Autodesk Fusion 360 part; units mm, degrees
(part 4 of 6)
extrude "Extrude2" cut sketch "Sketch2" against normal blind 2 contours L4 L5 L6 L7 A0 A1 A2 A3 | A4 L10 L11 A5 A6 L13 L14 A7 | A8 L16 L17 A9 A10 L19 L20 A11 | A12 L22 L23 A13 A14 L25 L26 A15 | A16 L28 L29 A17 A18 L31 L32 A19 | A20 L34 L35 A21 A22 L37 L38 A23 | A24 L40 L41 A25 A26 L43 L44 A27 | A28 L46 L47 A29 A30 L49 L50 A31 | A32 L52 L53 A33 A34 L55 L56 A35 | A36 L58 L59 A37 A38 L61 L62 A39 | A40 L64 L65 A41 A42 L67 L68 A43 | A44 L70 L71 A45 A46 L73 L74 A47 | A48 L76 L77 A49 A50 L79 L80 A51 | A52 L82 L83 A53 A54 L85 L86 A55 | A56 L88 L89 A57 A58 L91 L92 A59 | A60 L94 L95 A61 A62 L97 L98 A63 | A64 L100 L101 A65 A66 L103 L104 A67 | A68 L106 L107 A69 A70 L109 L110 A71 | A72 L112 L113 A73 A74 L115 L116 A75 | A76 L118 L119 A77 A78 L121 L122 A79 | A80 L124 L125 A81 A82 L127 L128 A83 | A84 L130 L131 A85 A86 L133 L134 A87 | A88 L136 L137 A89 A90 L139 L140 A91 | A92 L142 L143 A93 A94 L145 L146 A95 | A96 L148 L149 A97 A98 L151 L152 A99 | A100 L154 L155 A101 A102 L157 L158 A103 | A104 L160 L161 A105 A106 L163 L164 A107 | A108 L166 L167 A109 A110 L169 L170 A111 | A112 L172 L173 A113 A114 L175 L176 A115 | A116 L178 L179 A117 A118 L181 L182 A119 | A120 L184 L185 A121 A122 L187 L188 A123 | A124 L190 L191 A125 A126 L193 L194 A127 | A128 L196 L197 A129 A130 L199 L200 A131 | A132 L202 L203 A133 A134 L205 L206 A135 | A136 L208 L209 A137 A138 L211 L212 A139 | A140 L214 L215 A141 A142 L217 L218 A143 | A144 L220 L221 A145 A146 L223 L224 A147 | A148 L226 L227 A149 A150 L229 L230 A151 | A152 L232 L233 A153 A154 L235 L236 A155 | A156 L238 L239 A157 A158 L241 L242 A159 | A160 L244 L245 A161 A162 L247 L248 A163 | A164 L250 L251 A165 A166 L253 L254 A167 | A168 L256 L257 A169 A170 L259 L260 A171 | A172 L262 L263 A173 A174 L265 L266 A175 | A176 L268 L269 A177 A178 L271 L272 A179 | A180 L274 L275 A181 A182 L277 L278 A183 | A184 L280 L281 A185 A186 L283 L284 A187 | A188 L286 L287 A189 A190 L289 L290 A191 | A192 L292 L293 A193 A194 L295 L296 A195 | A196 L298 L299 A197 A198 L301 L302 A199 | A200 L304 L305 A201 A202 L307 L308 A203 | A204 L310 L311 A205 A206 L313 L314 A207 | A208 L316 L317 A209 A210 L319 L320 A211 | A212 L322 L323 A213 A214 L325 L326 A215 | A216 L328 L329 A217 A218 L331 L332 A219 | A220 L334 L335 A221 A222 L337 L338 A223 | A224 L340 L341 A225 A226 L343 L344 A227 | A228 L346 L347 A229 A230 L349 L350 A231 | A232 L352 L353 A233 A234 L355 L356 A235 | A236 L358 L359 A237 A238 L361 L362 A239 | A240 L364 L365 A241 A242 L367 L368 A243 | A244 L370 L371 A245 A246 L373 L374 A247 | A248 L376 L377 A249 A250 L379 L380 A251 | A252 L382 L383 A253 A254 L385 L386 A255 | A256 L388 L389 A257 A258 L391 L392 A259 | A260 L394 L395 A261 A262 L397 L398 A263 | A264 L400 L401 A265 A266 L403 L404 A267 | A268 L406 L407 A269 A270 L409 L410 A271 | A272 L412 L413 A273 A274 L415 L416 A275 | A276 L418 L419 A277 A278 L421 L422 A279 | A280 L424 L425 A281 A282 L427 L428 A283 | A284 L430 L431 A285 A286 L433 L434 A287 | A288 L436 L437 A289 A290 L439 L440 A291 | A292 L442 L443 A293 A294 L445 L446 A295 | A296 L448 L449 A297 A298 L451 L452 A299 | A300 L454 L455 A301 A302 L457 L458 A303 | A304 L460 L461 A305 A306 L463 L464 A307 | A308 L466 L467 A309 A310 L469 L470 A311 | A312 L472 L473 A313 A314 L475 L476 A315 | A316 L478 L479 A317 A318 L481 L482 A319 | A320 L484 L485 A321 A322 L487 L488 A323 | A324 L490 L491 A325 A326 L493 L494 A327 | A328 L496 L497 A329 A330 L499 L500 A331 | A332 L502 L503 A333 A334 L505 L506 A335 | A336 L508 L509 A337 A338 L511 L512 A339 | A340 L514 L515 A341 A342 L517 L518 A343 | A344 L520 L521 A345 A346 L523 L524 A347 | A348 L526 L527 A349 A350 L529 L530 A351 | A352 L532 L533 A353 A354 L535 L536 A355 | A356 L538 L539 A357 A358 L541 L542 A359 | A360 L544 L545 A361 A362 L547 L548 A363 | A364 L550 L551 A365 A366 L553 L554 A367 | A368 L556 L557 A369 A370 L559 L560 A371 | A372 L562 L563 A373 A374 L565 L566 A375 | A376 L568 L569 A377 A378 L571 L572 A379 | A380 L574 L575 A381 A382 L577 L578 A383 | A384 L580 L581 A385 A386 L583 L584 A387 | A388 L586 L587 A389 A390 L589 L590 A391 | A392 L592 L593 A393 A394 L595 L596 A395 | A396 L598 L599 A397 A398 L601 L602 A399 | A400 L604 L605 A401 A402 L607 L608 A403 | A404 L610 L611 A405 A406 L613 L614 A407 | A408 L616 L617 A409 A410 L619 L620 A411 | A412 L622 L623 A413 A414 L625 L626 A415 | A416 L628 L629 A417 A418 L631 L632 A419 | A420 L634 L635 A421 A422 L637 L638 A423 | A424 L640 L641 A425 A426 L643 L644 A427 | A428 L646 L647 A429 A430 L649 L650 A431 | A432 L652 L653 A433 A434 L655 L656 A435 | A436 L658 L659 A437 A438 L661 L662 A439 | A440 L664 L665 A441 A442 L667 L668 A443 | A444 L670 L671 A445 A446 L673 L674 A447 | A448 L676 L677 A449 A450 L679 L680 A451 | A452 L682 L683 A453 A454 L685 L686 A455 | A456 L688 L689 A457 A458 L691 L692 A459 | A460 L694 L695 A461 A462 L697 L698 A463 | A464 L700 L701 A465 A466 L703 L704 A467 | A468 L706 L707 A469 A470 L709 L710 A471 | A472 L712 L713 A473 A474 L715 L716 A475 | A476 L718 L719 A477 A478 L721 L722 A479 | A480 L724 L725 A481 A482 L727 L728 A483 | A484 L730 L731 A485 A486 L733 L734 A487 | A488 L736 L737 A489 A490 L739 L740 A491 | A492 L742 L743 A493 A494 L745 L746 A495 | A496 L748 L749 A497 A498 L751 L752 A499 | A500 L754 L755 A501 A502 L757 L758 A503 | A504 L760 L761 A505 A506 L763 L764 A507 | A508 L766 L767 A509 A510 L769 L770 A511 | A512 L772 L773 A513 A514 L775 L776 A515 | A516 L778 L779 A517 A518 L781 L782 A519 | A520 L784 L785 A521 A522 L787 L788 A523 | A524 L790 L791 A525 A526 L793 L794 A527 | A528 L796 L797 A529 A530 L799 L800 A531 | A532 L802 L803 A533 A534 L805 L806 A535 | A536 L808 L809 A537 A538 L811 L812 A539 | A540 L814 L815 A541 A542 L817 L818 A543 | A544 L820 L821 A545 A546 L823 L824 A547 | A548 L826 L827 A549 A550 L829 L830 A551 | A552 L832 L833 A553 A554 L835 L836 A555 | A556 L838 L839 A557 A558 L841 L842 A559 | A560 L844 L845 A561 A562 L847 L848 A563 | A564 L850 L851 A565 A566 L853 L854 A567 | A568 L856 L857 A569 A570 L859 L860 A571 | A572 L862 L863 A573 A574 L865 L866 A575 | A576 L868 L869 A577 A578 L871 L872 A579 | A580 L874 L875 A581 A582 L877 L878 A583 | A584 L880 L881 A585 A586 L883 L884 A587 | A588 L886 L887 A589 A590 L889 L890 A591 | A592 L892 L893 A593 A594 L895 L896 A595 | A596 L898 L899 A597 A598 L901 L902 A599 | A600 L904 L905 A601 A602 L907 L908 A603 | A604 L910 L911 A605 A606 L913 L914 A607 | A608 L916 L917 A609 A610 L919 L920 A611 | A612 L922 L923 A613 A614 L925 L926 A615 | A616 L928 L929 A617 A618 L931 L932 A619 | A620 L934 L935 A621 A622 L937 L938 A623 | A624 L940 L941 A625 A626 L943 L944 A627 | A628 L946 L947 A629 A630 L949 L950 A631 | A632 L952 L953 A633 A634 L955 L956 A635 | A636 L958 L959 A637 A638 L961 L962 A639 | A640 L964 L965 A641 A642 L967 L968 A643 | A644 L970 L971 A645 A646 L973 L974 A647 | A648 L976 L977 A649 A650 L979 L980 A651 | A652 L982 L983 A653 A654 L985 L986 A655 | A656 L988 L989 A657 A658 L991 L992 A659 | A660 L994 L995 A661 A662 L997 L998 A663 | A664 L1000 L1001 A665 A666 L1003 L1004 A667 | A668 L1006 L1007 A669 A670 L1009 L1010 A671 | A672 L1012 L1013 A673 A674 L1015 L1016 A675 | A676 L1018 L1019 A677 A678 L1021 L1022 A679 | A680 L1024 L1025 A681 A682 L1027 L1028 A683 | A684 L1030 L1031 A685 A686 L1033 L1034 A687 | A688 L1036 L1037 A689 A690 L1039 L1040 A691 | A692 L1042 L1043 A693 A694 L1045 L1046 A695 | A696 L1048 L1049 A697 A698 L1051 L1052 A699 | A700 L1054 L1055 A701 A702 L1057 L1058 A703 | A704 L1060 L1061 A705 A706 L1063 L1064 A707 | A708 L1066 L1067 A709 A710 L1069 L1070 A711 | A712 L1072 L1073 A713 A714 L1075 L1076 A715 | A716 L1078 L1079 A717 A718 L1081 L1082 A719 | A720 L1084 L1085 A721 A722 L1087 L1088 A723 | A724 L1090 L1091 A725 A726 L1093 L1094 A727 | A728 L1096 L1097 A729 A730 L1099 L1100 A731 | A732 L1102 L1103 A733 A734 L1105 L1106 A735 | A736 L1108 L1109 A737 A738 L1111 L1112 A739 | A740 L1114 L1115 A741 A742 L1117 L1118 A743 | A744 L1120 L1121 A745 A746 L1123 L1124 A747 | A748 L1126 L1127 A749 A750 L1129 L1130 A751 | A752 L1132 L1133 A753 A754 L1135 L1136 A755 | A756 L1138 L1139 A757 A758 L1141 L1142 A759 | A760 L1144 L1145 A761 A762 L1147 L1148 A763 | A764 L1150 L1151 A765 A766 L1153 L1154 A767 | A768 L1156 L1157 A769 A770 L1159 L1160 A771 | A772 L1162 L1163 A773 A774 L1165 L1166 A775 | A776 L1168 L1169 A777 A778 L1171 L1172 A779 | A780 L1174 L1175 A781 A782 L1177 L1178 A783 | A784 L1180 L1181 A785 A786 L1183 L1184 A787 | A788 L1186 L1187 A789 A790 L1189 L1190 A791 | A792 L1192 L1193 A793 A794 L1195 L1196 A795 | A796 L1198 L1199 A797 A798 L1201 L1202 A799 | A800 L1204 L1205 A801 A802 L1207 L1208 A803 | A804 L1210 L1211 A805 A806 L1213 L1214 A807 | A808 L1216 L1217 A809 A810 L1219 L1220 A811 | A812 L1222 L1223 A813 A814 L1225 L1226 A815 | A816 L1228 L1229 A817 A818 L1231 L1232 A819 | A820 L1234 L1235 A821 A822 L1237 L1238 A823 | A824 L1240 L1241 A825 A826 L1243 L1244 A827 | A828 L1246 L1247 A829 A830 L1249 L1250 A831 | A832 L1252 L1253 A833 A834 L1255 L1256 A835 | A836 L1258 L1259 A837 A838 L1261 L1262 A839 | A840 L1264 L1265 A841 A842 L1267 L1268 A843 | A844 L1270 L1271 A845 A846 L1273 L1274 A847 | A848 L1276 L1277 A849 A850 L1279 L1280 A851 | A852 L1282 L1283 A853 A854 L1285 L1286 A855 | A856 L1288 L1289 A857 A858 L1291 L1292 A859 | A860 L1294 L1295 A861 A862 L1297 L1298 A863 | A864 L1300 L1301 A865 A866 L1303 L1304 A867 | A868 L1306 L1307 A869 A870 L1309 L1310 A871 | A872 L1312 L1313 A873 A874 L1315 L1316 A875 | A876 L1318 L1319 A877 A878 L1321 L1322 A879 | A880 L1324 L1325 A881 A882 L1327 L1328 A883 | A884 L1330 L1331 A885 A886 L1333 L1334 A887 | A888 L1336 L1337 A889 A890 L1339 L1340 A891 | A892 L1342 L1343 A893 A894 L1345 L1346 A895 | A896 L1348 L1349 A897 A898 L1351 L1352 A899
fillet "Fillet1" radius 20 4 edges at (-254, 20.5994, 0) (0, 20.5994, -254) (254, 20.5994, 0) (0, 20.5994, 254)
extrude "Extrude3" cut 4 faces at (-165.8917, 18.5994, 164.8333) (-165.8917, 18.5994, -166.95) (165.8917, 18.5994, -164.8333) (164.8333, 18.5994, 165.8917) along direction (0, -1, 0) blind 3
extrude "Extrude4" cut 13 faces at (-98.1083, 18.5994, 164.8333) (2.1083, 18.5994, 164.8333) (93.8917, 18.5994, 164.8333) (164.8333, 18.5994, 93.8917) (164.8333, 18.5994, -2.1083) (164.8333, 18.5994, -98.1083) (93.8917, 18.5994, -171.1667) (-2.1083, 18.5994, -171.1667) (-98.1083, 18.5994, -171.1667) (-164.8333, 18.5994, -98.1083) (-164.8333, 18.5994, -2.1083) (-164.8333, 18.5994, 93.8917) (2.1083, 18.5994, -3.1667) along direction (0, -1, 0) blind 3
extrude "Extrude5" cut 12 faces at (-146.1083, 18.5994, -140.8333) (-118.95, 18.5994, -122.1083) (-97.05, 18.5994, -93.8917) (-69.8917, 18.5994, -75.1667) (-44.8333, 18.5994, -50.1083) (-25.05, 18.5994, -26.1083) (27.1667, 18.5994, 21.8917) (45.8917, 18.5994, 49.05) (73.05, 18.5994, 74.1083) (98.1083, 18.5994, 97.05) (122.1083, 18.5994, 116.8333) (141.8917, 18.5994, 147.1667) along direction (0, -1, 0) blind 3
extrude "Extrude6" cut 12 faces at (141.8917, 18.5994, -140.8333) (123.1667, 18.5994, -117.8917) (93.8917, 18.5994, -94.95) (73.05, 18.5994, -74.1083) (52.225, 18.5994, -51.1667) (27.1667, 18.5994, -26.1083) (-26.1083, 18.5994, 22.95) (-45.8917, 18.5994, 44.8333) (-75.1667, 18.5994, 74.1083) (-98.1083, 18.5994, 97.05) (-118.95, 18.5994, 117.8917) (-146.1083, 18.5994, 147.1667) along direction (0, -1, 0) blind 3
extrude "Extrude7" cut 20 faces at (147.1667, 18.5994, 45.8917) (123.1667, 18.5994, 26.1083) (98.1083, 18.5994, 3.1667) (123.1667, 18.5994, -21.8917) (147.1667, 18.5994, -50.1083) (3.1667, 18.5994, 93.8917) (-20.8333, 18.5994, 117.8917) (-45.8917, 18.5994, 140.8333) (20.8333, 18.5994, 122.1083) (50.1083, 18.5994, 140.8333) (-98.1083, 18.5994, 3.1667) (-117.8917, 18.5994, 27.1667) (-140.8333, 18.5994, 45.8917) (-118.95, 18.5994, -21.8917) (-140.8333, 18.5994, -50.1083) (3.1667, 18.5994, -98.1083) (20.8333, 18.5994, -117.8917) (50.1083, 18.5994, -147.1667) (-20.8333, 18.5994, -122.1083) (-45.8917, 18.5994, -147.1667) along direction (0, -1, 0) blind 3
sketch "Sketch5" plane through (0, 20.5994, 0) normal (0, 1, 0) x (-1, 0, 0)
  line L0 (110.5, -150.325) -> (110.5, -137.675)
  arc A0 (113.675, -134.5) -> (110.5, -137.675) centre (113.675, -137.675) ccw
  line L1 (113.675, -134.5) -> (126.325, -134.5)
  arc A1 (129.5, -137.675) -> (126.325, -134.5) centre (126.325, -137.675) ccw
  line L2 (129.5, -137.675) -> (129.5, -150.325)
  arc A2 (126.325, -153.5) -> (129.5, -150.325) centre (126.325, -150.325) ccw
  line L3 (126.325, -153.5) -> (113.675, -153.5)
  arc A3 (110.5, -150.325) -> (113.675, -153.5) centre (113.675, -150.325) ccw
  line L4 (-9.5, -78.325) -> (-9.5, -65.675)
  arc A4 (-6.325, -62.5) -> (-9.5, -65.675) centre (-6.325, -65.675) ccw
  line L5 (-6.325, -62.5) -> (6.325, -62.5)
  arc A5 (9.5, -65.675) -> (6.325, -62.5) centre (6.325, -65.675) ccw
  line L6 (9.5, -65.675) -> (9.5, -78.325)
  arc A6 (6.325, -81.5) -> (9.5, -78.325) centre (6.325, -78.325) ccw
  line L7 (6.325, -81.5) -> (-6.325, -81.5)
  arc A7 (-9.5, -78.325) -> (-6.325, -81.5) centre (-6.325, -78.325) ccw
  line L8 (-153.5, 41.675) -> (-153.5, 54.325)
  arc A8 (-150.325, 57.5) -> (-153.5, 54.325) centre (-150.325, 54.325) ccw
  line L9 (-150.325, 57.5) -> (-137.675, 57.5)
  arc A9 (-134.5, 54.325) -> (-137.675, 57.5) centre (-137.675, 54.325) ccw
  line L10 (-134.5, 54.325) -> (-134.5, 41.675)
  arc A10 (-137.675, 38.5) -> (-134.5, 41.675) centre (-137.675, 41.675) ccw
  line L11 (-137.675, 38.5) -> (-150.325, 38.5)
  arc A11 (-153.5, 41.675) -> (-150.325, 38.5) centre (-150.325, 41.675) ccw
  line L12 (-81.5, -150.325) -> (-81.5, -137.675)
  arc A12 (-78.325, -134.5) -> (-81.5, -137.675) centre (-78.325, -137.675) ccw
  line L13 (-78.325, -134.5) -> (-65.675, -134.5)
  arc A13 (-62.5, -137.675) -> (-65.675, -134.5) centre (-65.675, -137.675) ccw
  line L14 (-62.5, -137.675) -> (-62.5, -150.325)
  arc A14 (-65.675, -153.5) -> (-62.5, -150.325) centre (-65.675, -150.325) ccw
  line L15 (-65.675, -153.5) -> (-78.325, -153.5)
  arc A15 (-81.5, -150.325) -> (-78.325, -153.5) centre (-78.325, -150.325) ccw
  line L16 (-33.5, -174.325) -> (-33.5, -161.675)
  arc A16 (-30.325, -158.5) -> (-33.5, -161.675) centre (-30.325, -161.675) ccw
  line L17 (-30.325, -158.5) -> (-17.675, -158.5)
  arc A17 (-14.5, -161.675) -> (-17.675, -158.5) centre (-17.675, -161.675) ccw
  line L18 (-14.5, -161.675) -> (-14.5, -174.325)
  arc A18 (-17.675, -177.5) -> (-14.5, -174.325) centre (-17.675, -174.325) ccw
  line L19 (-17.675, -177.5) -> (-30.325, -177.5)
  arc A19 (-33.5, -174.325) -> (-30.325, -177.5) centre (-30.325, -174.325) ccw
  line L20 (38.5, -126.325) -> (38.5, -113.675)
  arc A20 (41.675, -110.5) -> (38.5, -113.675) centre (41.675, -113.675) ccw
  line L21 (41.675, -110.5) -> (54.325, -110.5)
  arc A21 (57.5, -113.675) -> (54.325, -110.5) centre (54.325, -113.675) ccw
  line L22 (57.5, -113.675) -> (57.5, -126.325)
  arc A22 (54.325, -129.5) -> (57.5, -126.325) centre (54.325, -126.325) ccw
  line L23 (54.325, -129.5) -> (41.675, -129.5)
  arc A23 (38.5, -126.325) -> (41.675, -129.5) centre (41.675, -126.325) ccw
  line L24 (62.5, -150.325) -> (62.5, -137.675)
  arc A24 (65.675, -134.5) -> (62.5, -137.675) centre (65.675, -137.675) ccw
  line L25 (65.675, -134.5) -> (78.325, -134.5)
  arc A25 (81.5, -137.675) -> (78.325, -134.5) centre (78.325, -137.675) ccw
  line L26 (81.5, -137.675) -> (81.5, -150.325)
  arc A26 (78.325, -153.5) -> (81.5, -150.325) centre (78.325, -150.325) ccw
  line L27 (78.325, -153.5) -> (65.675, -153.5)
  arc A27 (62.5, -150.325) -> (65.675, -153.5) centre (65.675, -150.325) ccw
  line L28 (134.5, -102.325) -> (134.5, -89.675)
  arc A28 (137.675, -86.5) -> (134.5, -89.675) centre (137.675, -89.675) ccw
  line L29 (137.675, -86.5) -> (150.325, -86.5)
  arc A29 (153.5, -89.675) -> (150.325, -86.5) centre (150.325, -89.675) ccw
  line L30 (153.5, -89.675) -> (153.5, -102.325)
  arc A30 (150.325, -105.5) -> (153.5, -102.325) centre (150.325, -102.325) ccw
  line L31 (150.325, -105.5) -> (137.675, -105.5)
  arc A31 (134.5, -102.325) -> (137.675, -105.5) centre (137.675, -102.325) ccw
  line L32 (-33.5, -6.325) -> (-33.5, 6.325)
  arc A32 (-30.325, 9.5) -> (-33.5, 6.325) centre (-30.325, 6.325) ccw
  line L33 (-30.325, 9.5) -> (-17.675, 9.5)
  arc A33 (-14.5, 6.325) -> (-17.675, 9.5) centre (-17.675, 6.325) ccw
  line L34 (-14.5, 6.325) -> (-14.5, -6.325)
  arc A34 (-17.675, -9.5) -> (-14.5, -6.325) centre (-17.675, -6.325) ccw
  line L35 (-17.675, -9.5) -> (-30.325, -9.5)
  arc A35 (-33.5, -6.325) -> (-30.325, -9.5) centre (-30.325, -6.325) ccw
  line L36 (-105.5, -174.325) -> (-105.5, -161.675)
  arc A36 (-102.325, -158.5) -> (-105.5, -161.675) centre (-102.325, -161.675) ccw
  line L37 (-102.325, -158.5) -> (-89.675, -158.5)
  arc A37 (-86.5, -161.675) -> (-89.675, -158.5) centre (-89.675, -161.675) ccw
  line L38 (-86.5, -161.675) -> (-86.5, -174.325)
  arc A38 (-89.675, -177.5) -> (-86.5, -174.325) centre (-89.675, -174.325) ccw
  line L39 (-89.675, -177.5) -> (-102.325, -177.5)
  arc A39 (-105.5, -174.325) -> (-102.325, -177.5) centre (-102.325, -174.325) ccw
  line L40 (-81.5, -30.325) -> (-81.5, -17.675)
  arc A40 (-78.325, -14.5) -> (-81.5, -17.675) centre (-78.325, -17.675) ccw
  line L41 (-78.325, -14.5) -> (-65.675, -14.5)
  arc A41 (-62.5, -17.675) -> (-65.675, -14.5) centre (-65.675, -17.675) ccw
  line L42 (-62.5, -17.675) -> (-62.5, -30.325)
  arc A42 (-65.675, -33.5) -> (-62.5, -30.325) centre (-65.675, -30.325) ccw
  line L43 (-65.675, -33.5) -> (-78.325, -33.5)
  arc A43 (-81.5, -30.325) -> (-78.325, -33.5) centre (-78.325, -30.325) ccw
  line L44 (134.5, -174.325) -> (134.5, -161.675)
  arc A44 (137.675, -158.5) -> (134.5, -161.675) centre (137.675, -161.675) ccw
  line L45 (137.675, -158.5) -> (150.325, -158.5)
  arc A45 (153.5, -161.675) -> (150.325, -158.5) centre (150.325, -161.675) ccw
  line L46 (153.5, -161.675) -> (153.5, -174.325)
  arc A46 (150.325, -177.5) -> (153.5, -174.325) centre (150.325, -174.325) ccw
  line L47 (150.325, -177.5) -> (137.675, -177.5)
  arc A47 (134.5, -174.325) -> (137.675, -177.5) centre (137.675, -174.325) ccw
  line L48 (158.5, -150.325) -> (158.5, -137.675)
  arc A48 (161.675, -134.5) -> (158.5, -137.675) centre (161.675, -137.675) ccw
  line L49 (161.675, -134.5) -> (174.325, -134.5)
  arc A49 (177.5, -137.675) -> (174.325, -134.5) centre (174.325, -137.675) ccw
  line L50 (177.5, -137.675) -> (177.5, -150.325)
  arc A50 (174.325, -153.5) -> (177.5, -150.325) centre (174.325, -150.325) ccw
  line L51 (174.325, -153.5) -> (161.675, -153.5)
  arc A51 (158.5, -150.325) -> (161.675, -153.5) centre (161.675, -150.325) ccw
  line L52 (110.5, -78.325) -> (110.5, -65.675)
  arc A52 (113.675, -62.5) -> (110.5, -65.675) centre (113.675, -65.675) ccw
  line L53 (113.675, -62.5) -> (126.325, -62.5)
  arc A53 (129.5, -65.675) -> (126.325, -62.5) centre (126.325, -65.675) ccw
  line L54 (129.5, -65.675) -> (129.5, -78.325)
  arc A54 (126.325, -81.5) -> (129.5, -78.325) centre (126.325, -78.325) ccw
  line L55 (126.325, -81.5) -> (113.675, -81.5)
  arc A55 (110.5, -78.325) -> (113.675, -81.5) centre (113.675, -78.325) ccw
  line L56 (62.5, -126.325) -> (62.5, -113.675)
  arc A56 (65.675, -110.5) -> (62.5, -113.675) centre (65.675, -113.675) ccw
  line L57 (65.675, -110.5) -> (78.325, -110.5)
  arc A57 (81.5, -113.675) -> (78.325, -110.5) centre (78.325, -113.675) ccw
  line L58 (81.5, -113.675) -> (81.5, -126.325)
  arc A58 (78.325, -129.5) -> (81.5, -126.325) centre (78.325, -126.325) ccw
  line L59 (78.325, -129.5) -> (65.675, -129.5)
  arc A59 (62.5, -126.325) -> (65.675, -129.5) centre (65.675, -126.325) ccw
  line L60 (62.5, -102.325) -> (62.5, -89.675)
  arc A60 (65.675, -86.5) -> (62.5, -89.675) centre (65.675, -89.675) ccw
  line L61 (65.675, -86.5) -> (78.325, -86.5)
  arc A61 (81.5, -89.675) -> (78.325, -86.5) centre (78.325, -89.675) ccw
  line L62 (81.5, -89.675) -> (81.5, -102.325)
  arc A62 (78.325, -105.5) -> (81.5, -102.325) centre (78.325, -102.325) ccw
  line L63 (78.325, -105.5) -> (65.675, -105.5)
  arc A63 (62.5, -102.325) -> (65.675, -105.5) centre (65.675, -102.325) ccw
  line L64 (14.5, -30.325) -> (14.5, -17.675)
  arc A64 (17.675, -14.5) -> (14.5, -17.675) centre (17.675, -17.675) ccw
  line L65 (17.675, -14.5) -> (30.325, -14.5)
  arc A65 (33.5, -17.675) -> (30.325, -14.5) centre (30.325, -17.675) ccw
  line L66 (33.5, -17.675) -> (33.5, -30.325)
  arc A66 (30.325, -33.5) -> (33.5, -30.325) centre (30.325, -30.325) ccw
  line L67 (30.325, -33.5) -> (17.675, -33.5)
  arc A67 (14.5, -30.325) -> (17.675, -33.5) centre (17.675, -30.325) ccw
  line L68 (110.5, -6.325) -> (110.5, 6.325)
  arc A68 (113.675, 9.5) -> (110.5, 6.325) centre (113.675, 6.325) ccw
  line L69 (113.675, 9.5) -> (126.325, 9.5)
  arc A69 (129.5, 6.325) -> (126.325, 9.5) centre (126.325, 6.325) ccw
  line L70 (129.5, 6.325) -> (129.5, -6.325)
  arc A70 (126.325, -9.5) -> (129.5, -6.325) centre (126.325, -6.325) ccw
  line L71 (126.325, -9.5) -> (113.675, -9.5)
  arc A71 (110.5, -6.325) -> (113.675, -9.5) centre (113.675, -6.325) ccw
  line L72 (110.5, 17.675) -> (110.5, 30.325)
  arc A72 (113.675, 33.5) -> (110.5, 30.325) centre (113.675, 30.325) ccw
  line L73 (113.675, 33.5) -> (126.325, 33.5)
  arc A73 (129.5, 30.325) -> (126.325, 33.5) centre (126.325, 30.325) ccw
  line L74 (129.5, 30.325) -> (129.5, 17.675)
  arc A74 (126.325, 14.5) -> (129.5, 17.675) centre (126.325, 17.675) ccw
  line L75 (126.325, 14.5) -> (113.675, 14.5)
  arc A75 (110.5, 17.675) -> (113.675, 14.5) centre (113.675, 17.675) ccw
  line L76 (110.5, 41.675) -> (110.5, 54.325)
  arc A76 (113.675, 57.5) -> (110.5, 54.325) centre (113.675, 54.325) ccw
  line L77 (113.675, 57.5) -> (126.325, 57.5)
  arc A77 (129.5, 54.325) -> (126.325, 57.5) centre (126.325, 54.325) ccw
  line L78 (129.5, 54.325) -> (129.5, 41.675)
  arc A78 (126.325, 38.5) -> (129.5, 41.675) centre (126.325, 41.675) ccw
  line L79 (126.325, 38.5) -> (113.675, 38.5)
  arc A79 (110.5, 41.675) -> (113.675, 38.5) centre (113.675, 41.675) ccw
  line L80 (110.5, 65.675) -> (110.5, 78.325)
  arc A80 (113.675, 81.5) -> (110.5, 78.325) centre (113.675, 78.325) ccw
  line L81 (113.675, 81.5) -> (126.325, 81.5)
  arc A81 (129.5, 78.325) -> (126.325, 81.5) centre (126.325, 78.325) ccw
  line L82 (129.5, 78.325) -> (129.5, 65.675)
  arc A82 (126.325, 62.5) -> (129.5, 65.675) centre (126.325, 65.675) ccw
  line L83 (126.325, 62.5) -> (113.675, 62.5)
  arc A83 (110.5, 65.675) -> (113.675, 62.5) centre (113.675, 65.675) ccw
  line L84 (110.5, 89.675) -> (110.5, 102.325)
  arc A84 (113.675, 105.5) -> (110.5, 102.325) centre (113.675, 102.325) ccw
  line L85 (113.675, 105.5) -> (126.325, 105.5)
  arc A85 (129.5, 102.325) -> (126.325, 105.5) centre (126.325, 102.325) ccw
  line L86 (129.5, 102.325) -> (129.5, 89.675)
  arc A86 (126.325, 86.5) -> (129.5, 89.675) centre (126.325, 89.675) ccw
  line L87 (126.325, 86.5) -> (113.675, 86.5)
  arc A87 (110.5, 89.675) -> (113.675, 86.5) centre (113.675, 89.675) ccw
  line L88 (110.5, 113.675) -> (110.5, 126.325)
  arc A88 (113.675, 129.5) -> (110.5, 126.325) centre (113.675, 126.325) ccw
  line L89 (113.675, 129.5) -> (126.325, 129.5)
  arc A89 (129.5, 126.325) -> (126.325, 129.5) centre (126.325, 126.325) ccw
  line L90 (129.5, 126.325) -> (129.5, 113.675)
  arc A90 (126.325, 110.5) -> (129.5, 113.675) centre (126.325, 113.675) ccw
  line L91 (126.325, 110.5) -> (113.675, 110.5)
  arc A91 (110.5, 113.675) -> (113.675, 110.5) centre (113.675, 113.675) ccw
  line L92 (110.5, 137.675) -> (110.5, 150.325)
  arc A92 (113.675, 153.5) -> (110.5, 150.325) centre (113.675, 150.325) ccw
  line L93 (113.675, 153.5) -> (126.325, 153.5)
  arc A93 (129.5, 150.325) -> (126.325, 153.5) centre (126.325, 150.325) ccw
  line L94 (129.5, 150.325) -> (129.5, 137.675)
  arc A94 (126.325, 134.5) -> (129.5, 137.675) centre (126.325, 137.675) ccw
  line L95 (126.325, 134.5) -> (113.675, 134.5)
  arc A95 (110.5, 137.675) -> (113.675, 134.5) centre (113.675, 137.675) ccw
  line L96 (110.5, 161.675) -> (110.5, 174.325)
  arc A96 (113.675, 177.5) -> (110.5, 174.325) centre (113.675, 174.325) ccw
  line L97 (113.675, 177.5) -> (126.325, 177.5)
  arc A97 (129.5, 174.325) -> (126.325, 177.5) centre (126.325, 174.325) ccw
  line L98 (129.5, 174.325) -> (129.5, 161.675)
  arc A98 (126.325, 158.5) -> (129.5, 161.675) centre (126.325, 161.675) ccw
  line L99 (126.325, 158.5) -> (113.675, 158.5)
  arc A99 (110.5, 161.675) -> (113.675, 158.5) centre (113.675, 161.675) ccw
  line L100 (38.5, -6.325) -> (38.5, 6.325)
  arc A100 (41.675, 9.5) -> (38.5, 6.325) centre (41.675, 6.325) ccw
  line L101 (41.675, 9.5) -> (54.325, 9.5)
  arc A101 (57.5, 6.325) -> (54.325, 9.5) centre (54.325, 6.325) ccw
  line L102 (57.5, 6.325) -> (57.5, -6.325)
  arc A102 (54.325, -9.5) -> (57.5, -6.325) centre (54.325, -6.325) ccw
  line L103 (54.325, -9.5) -> (41.675, -9.5)
  arc A103 (38.5, -6.325) -> (41.675, -9.5) centre (41.675, -6.325) ccw
  line L104 (38.5, 17.675) -> (38.5, 30.325)
  arc A104 (41.675, 33.5) -> (38.5, 30.325) centre (41.675, 30.325) ccw
  line L105 (41.675, 33.5) -> (54.325, 33.5)
  arc A105 (57.5, 30.325) -> (54.325, 33.5) centre (54.325, 30.325) ccw
  line L106 (57.5, 30.325) -> (57.5, 17.675)
  arc A106 (54.325, 14.5) -> (57.5, 17.675) centre (54.325, 17.675) ccw
  line L107 (54.325, 14.5) -> (41.675, 14.5)
  arc A107 (38.5, 17.675) -> (41.675, 14.5) centre (41.675, 17.675) ccw
  line L108 (38.5, 41.675) -> (38.5, 54.325)
  arc A108 (41.675, 57.5) -> (38.5, 54.325) centre (41.675, 54.325) ccw
  line L109 (41.675, 57.5) -> (54.325, 57.5)
  arc A109 (57.5, 54.325) -> (54.325, 57.5) centre (54.325, 54.325) ccw
  line L110 (57.5, 54.325) -> (57.5, 41.675)
  arc A110 (54.325, 38.5) -> (57.5, 41.675) centre (54.325, 41.675) ccw
  line L111 (54.325, 38.5) -> (41.675, 38.5)
  arc A111 (38.5, 41.675) -> (41.675, 38.5) centre (41.675, 41.675) ccw
  line L112 (38.5, 65.675) -> (38.5, 78.325)
  arc A112 (41.675, 81.5) -> (38.5, 78.325) centre (41.675, 78.325) ccw
  line L113 (41.675, 81.5) -> (54.325, 81.5)
  arc A113 (57.5, 78.325) -> (54.325, 81.5) centre (54.325, 78.325) ccw
  line L114 (57.5, 78.325) -> (57.5, 65.675)
  arc A114 (54.325, 62.5) -> (57.5, 65.675) centre (54.325, 65.675) ccw
  line L115 (54.325, 62.5) -> (41.675, 62.5)
  arc A115 (38.5, 65.675) -> (41.675, 62.5) centre (41.675, 65.675) ccw
  line L116 (14.5, 89.675) -> (14.5, 102.325)
  arc A116 (17.675, 105.5) -> (14.5, 102.325) centre (17.675, 102.325) ccw
  line L117 (17.675, 105.5) -> (30.325, 105.5)
  arc A117 (33.5, 102.325) -> (30.325, 105.5) centre (30.325, 102.325) ccw
  line L118 (33.5, 102.325) -> (33.5, 89.675)
  arc A118 (30.325, 86.5) -> (33.5, 89.675) centre (30.325, 89.675) ccw
  line L119 (30.325, 86.5) -> (17.675, 86.5)
  arc A119 (14.5, 89.675) -> (17.675, 86.5) centre (17.675, 89.675) ccw
  line L120 (14.5, 113.675) -> (14.5, 126.325)
  arc A120 (17.675, 129.5) -> (14.5, 126.325) centre (17.675, 126.325) ccw
  line L121 (17.675, 129.5) -> (30.325, 129.5)
  arc A121 (33.5, 126.325) -> (30.325, 129.5) centre (30.325, 126.325) ccw
  line L122 (33.5, 126.325) -> (33.5, 113.675)
  arc A122 (30.325, 110.5) -> (33.5, 113.675) centre (30.325, 113.675) ccw
  line L123 (30.325, 110.5) -> (17.675, 110.5)
  arc A123 (14.5, 113.675) -> (17.675, 110.5) centre (17.675, 113.675) ccw
  line L124 (14.5, 137.675) -> (14.5, 150.325)
  arc A124 (17.675, 153.5) -> (14.5, 150.325) centre (17.675, 150.325) ccw
  line L125 (17.675, 153.5) -> (30.325, 153.5)
  arc A125 (33.5, 150.325) -> (30.325, 153.5) centre (30.325, 150.325) ccw
  line L126 (33.5, 150.325) -> (33.5, 137.675)
  arc A126 (30.325, 134.5) -> (33.5, 137.675) centre (30.325, 137.675) ccw
  line L127 (30.325, 134.5) -> (17.675, 134.5)
  arc A127 (14.5, 137.675) -> (17.675, 134.5) centre (17.675, 137.675) ccw
  line L128 (-9.5, 161.675) -> (-9.5, 174.325)
  arc A128 (-6.325, 177.5) -> (-9.5, 174.325) centre (-6.325, 174.325) ccw
  line L129 (-6.325, 177.5) -> (6.325, 177.5)
  arc A129 (9.5, 174.325) -> (6.325, 177.5) centre (6.325, 174.325) ccw
  line L130 (9.5, 174.325) -> (9.5, 161.675)
  arc A130 (6.325, 158.5) -> (9.5, 161.675) centre (6.325, 161.675) ccw
  line L131 (6.325, 158.5) -> (-6.325, 158.5)
  arc A131 (-9.5, 161.675) -> (-6.325, 158.5) centre (-6.325, 161.675) ccw
  line L132 (-105.5, 17.675) -> (-105.5, 30.325)
  arc A132 (-102.325, 33.5) -> (-105.5, 30.325) centre (-102.325, 30.325) ccw
  line L133 (-102.325, 33.5) -> (-89.675, 33.5)
  arc A133 (-86.5, 30.325) -> (-89.675, 33.5) centre (-89.675, 30.325) ccw
  line L134 (-86.5, 30.325) -> (-86.5, 17.675)
  arc A134 (-89.675, 14.5) -> (-86.5, 17.675) centre (-89.675, 17.675) ccw
  line L135 (-89.675, 14.5) -> (-102.325, 14.5)
  arc A135 (-105.5, 17.675) -> (-102.325, 14.5) centre (-102.325, 17.675) ccw
  line L136 (-129.5, 41.675) -> (-129.5, 54.325)
  arc A136 (-126.325, 57.5) -> (-129.5, 54.325) centre (-126.325, 54.325) ccw
  line L137 (-126.325, 57.5) -> (-113.675, 57.5)
  arc A137 (-110.5, 54.325) -> (-113.675, 57.5) centre (-113.675, 54.325) ccw
  line L138 (-110.5, 54.325) -> (-110.5, 41.675)
  arc A138 (-113.675, 38.5) -> (-110.5, 41.675) centre (-113.675, 41.675) ccw
  line L139 (-113.675, 38.5) -> (-126.325, 38.5)
  arc A139 (-129.5, 41.675) -> (-126.325, 38.5) centre (-126.325, 41.675) ccw
  line L140 (-153.5, -30.325) -> (-153.5, -17.675)
  arc A140 (-150.325, -14.5) -> (-153.5, -17.675) centre (-150.325, -17.675) ccw
  line L141 (-150.325, -14.5) -> (-137.675, -14.5)
  arc A141 (-134.5, -17.675) -> (-137.675, -14.5) centre (-137.675, -17.675) ccw
  line L142 (-134.5, -17.675) -> (-134.5, -30.325)
  arc A142 (-137.675, -33.5) -> (-134.5, -30.325) centre (-137.675, -30.325) ccw
  line L143 (-137.675, -33.5) -> (-150.325, -33.5)
  arc A143 (-153.5, -30.325) -> (-150.325, -33.5) centre (-150.325, -30.325) ccw
  line L144 (-177.5, 17.675) -> (-177.5, 30.325)
  arc A144 (-174.325, 33.5) -> (-177.5, 30.325) centre (-174.325, 30.325) ccw
  line L145 (-174.325, 33.5) -> (-161.675, 33.5)
  arc A145 (-158.5, 30.325) -> (-161.675, 33.5) centre (-161.675, 30.325) ccw
  line L146 (-158.5, 30.325) -> (-158.5, 17.675)
  arc A146 (-161.675, 14.5) -> (-158.5, 17.675) centre (-161.675, 17.675) ccw
  line L147 (-161.675, 14.5) -> (-174.325, 14.5)
  arc A147 (-177.5, 17.675) -> (-174.325, 14.5) centre (-174.325, 17.675) ccw
  line L148 (-9.5, -174.325) -> (-9.5, -161.675)
  arc A148 (-6.325, -158.5) -> (-9.5, -161.675) centre (-6.325, -161.675) ccw
  line L149 (-6.325, -158.5) -> (6.325, -158.5)
  arc A149 (9.5, -161.675) -> (6.325, -158.5) centre (6.325, -161.675) ccw
  line L150 (9.5, -161.675) -> (9.5, -174.325)
  arc A150 (6.325, -177.5) -> (9.5, -174.325) centre (6.325, -174.325) ccw
  line L151 (6.325, -177.5) -> (-6.325, -177.5)
  arc A151 (-9.5, -174.325) -> (-6.325, -177.5) centre (-6.325, -174.325) ccw
  line L152 (-33.5, -126.325) -> (-33.5, -113.675)
  arc A152 (-30.325, -110.5) -> (-33.5, -113.675) centre (-30.325, -113.675) ccw
  line L153 (-30.325, -110.5) -> (-17.675, -110.5)
  arc A153 (-14.5, -113.675) -> (-17.675, -110.5) centre (-17.675, -113.675) ccw
  line L154 (-14.5, -113.675) -> (-14.5, -126.325)
  arc A154 (-17.675, -129.5) -> (-14.5, -126.325) centre (-17.675, -126.325) ccw
  line L155 (-17.675, -129.5) -> (-30.325, -129.5)
  arc A155 (-33.5, -126.325) -> (-30.325, -129.5) centre (-30.325, -126.325) ccw
  line L156 (-81.5, -78.325) -> (-81.5, -65.675)
  arc A156 (-78.325, -62.5) -> (-81.5, -65.675) centre (-78.325, -65.675) ccw
  line L157 (-78.325, -62.5) -> (-65.675, -62.5)
  arc A157 (-62.5, -65.675) -> (-65.675, -62.5) centre (-65.675, -65.675) ccw
  line L158 (-62.5, -65.675) -> (-62.5, -78.325)
  arc A158 (-65.675, -81.5) -> (-62.5, -78.325) centre (-65.675, -78.325) ccw
  line L159 (-65.675, -81.5) -> (-78.325, -81.5)
  arc A159 (-81.5, -78.325) -> (-78.325, -81.5) centre (-78.325, -78.325) ccw
  line L160 (-153.5, -174.325) -> (-153.5, -161.675)
  arc A160 (-150.325, -158.5) -> (-153.5, -161.675) centre (-150.325, -161.675) ccw
  line L161 (-150.325, -158.5) -> (-137.675, -158.5)
  arc A161 (-134.5, -161.675) -> (-137.675, -158.5) centre (-137.675, -161.675) ccw
  line L162 (-134.5, -161.675) -> (-134.5, -174.325)
  arc A162 (-137.675, -177.5) -> (-134.5, -174.325) centre (-137.675, -174.325) ccw
  line L163 (-137.675, -177.5) -> (-150.325, -177.5)
  arc A163 (-153.5, -174.325) -> (-150.325, -177.5) centre (-150.325, -174.325) ccw
  line L164 (-129.5, -150.325) -> (-129.5, -137.675)
  arc A164 (-126.325, -134.5) -> (-129.5, -137.675) centre (-126.325, -137.675) ccw
  line L165 (-126.325, -134.5) -> (-113.675, -134.5)
  arc A165 (-110.5, -137.675) -> (-113.675, -134.5) centre (-113.675, -137.675) ccw
  line L166 (-110.5, -137.675) -> (-110.5, -150.325)
  arc A166 (-113.675, -153.5) -> (-110.5, -150.325) centre (-113.675, -150.325) ccw
  line L167 (-113.675, -153.5) -> (-126.325, -153.5)
  arc A167 (-129.5, -150.325) -> (-126.325, -153.5) centre (-126.325, -150.325) ccw
  line L168 (-177.5, -102.325) -> (-177.5, -89.675)
  arc A168 (-174.325, -86.5) -> (-177.5, -89.675) centre (-174.325, -89.675) ccw
  line L169 (-174.325, -86.5) -> (-161.675, -86.5)
  arc A169 (-158.5, -89.675) -> (-161.675, -86.5) centre (-161.675, -89.675) ccw
  line L170 (-158.5, -89.675) -> (-158.5, -102.325)
  arc A170 (-161.675, -105.5) -> (-158.5, -102.325) centre (-161.675, -102.325) ccw
  line L171 (-161.675, -105.5) -> (-174.325, -105.5)
  arc A171 (-177.5, -102.325) -> (-174.325, -105.5) centre (-174.325, -102.325) ccw
  line L172 (-153.5, -78.325) -> (-153.5, -65.675)
  arc A172 (-150.325, -62.5) -> (-153.5, -65.675) centre (-150.325, -65.675) ccw
  line L173 (-150.325, -62.5) -> (-137.675, -62.5)
  arc A173 (-134.5, -65.675) -> (-137.675, -62.5) centre (-137.675, -65.675) ccw
  line L174 (-134.5, -65.675) -> (-134.5, -78.325)
  arc A174 (-137.675, -81.5) -> (-134.5, -78.325) centre (-137.675, -78.325) ccw
  line L175 (-137.675, -81.5) -> (-150.325, -81.5)
  arc A175 (-153.5, -78.325) -> (-150.325, -81.5) centre (-150.325, -78.325) ccw
  line L176 (-33.5, 41.675) -> (-33.5, 54.325)
  arc A176 (-30.325, 57.5) -> (-33.5, 54.325) centre (-30.325, 54.325) ccw
  line L177 (-30.325, 57.5) -> (-17.675, 57.5)
  arc A177 (-14.5, 54.325) -> (-17.675, 57.5) centre (-17.675, 54.325) ccw
  line L178 (-14.5, 54.325) -> (-14.5, 41.675)
  arc A178 (-17.675, 38.5) -> (-14.5, 41.675) centre (-17.675, 41.675) ccw
  line L179 (-17.675, 38.5) -> (-30.325, 38.5)
  arc A179 (-33.5, 41.675) -> (-30.325, 38.5) centre (-30.325, 41.675) ccw
  line L180 (-105.5, 65.675) -> (-105.5, 78.325)
  arc A180 (-102.325, 81.5) -> (-105.5, 78.325) centre (-102.325, 78.325) ccw
  line L181 (-102.325, 81.5) -> (-89.675, 81.5)
  arc A181 (-86.5, 78.325) -> (-89.675, 81.5) centre (-89.675, 78.325) ccw
  line L182 (-86.5, 78.325) -> (-86.5, 65.675)
  arc A182 (-89.675, 62.5) -> (-86.5, 65.675) centre (-89.675, 65.675) ccw
  line L183 (-89.675, 62.5) -> (-102.325, 62.5)
  arc A183 (-105.5, 65.675) -> (-102.325, 62.5) centre (-102.325, 65.675) ccw
  line L184 (-177.5, 89.675) -> (-177.5, 102.325)
  arc A184 (-174.325, 105.5) -> (-177.5, 102.325) centre (-174.325, 102.325) ccw
  line L185 (-174.325, 105.5) -> (-161.675, 105.5)
  arc A185 (-158.5, 102.325) -> (-161.675, 105.5) centre (-161.675, 102.325) ccw
  line L186 (-158.5, 102.325) -> (-158.5, 89.675)
  arc A186 (-161.675, 86.5) -> (-158.5, 89.675) centre (-161.675, 89.675) ccw
  line L187 (-161.675, 86.5) -> (-174.325, 86.5)
  arc A187 (-177.5, 89.675) -> (-174.325, 86.5) centre (-174.325, 89.675) ccw
  line L188 (-81.5, 89.675) -> (-81.5, 102.325)
  arc A188 (-78.325, 105.5) -> (-81.5, 102.325) centre (-78.325, 102.325) ccw
  line L189 (-78.325, 105.5) -> (-65.675, 105.5)
  arc A189 (-62.5, 102.325) -> (-65.675, 105.5) centre (-65.675, 102.325) ccw
  line L190 (-62.5, 102.325) -> (-62.5, 89.675)
  arc A190 (-65.675, 86.5) -> (-62.5, 89.675) centre (-65.675, 89.675) ccw
  line L191 (-65.675, 86.5) -> (-78.325, 86.5)
  arc A191 (-81.5, 89.675) -> (-78.325, 86.5) centre (-78.325, 89.675) ccw
  line L192 (-153.5, 113.675) -> (-153.5, 126.325)
  arc A192 (-150.325, 129.5) -> (-153.5, 126.325) centre (-150.325, 126.325) ccw
  line L193 (-150.325, 129.5) -> (-137.675, 129.5)
  arc A193 (-134.5, 126.325) -> (-137.675, 129.5) centre (-137.675, 126.325) ccw
  line L194 (-134.5, 126.325) -> (-134.5, 113.675)
  arc A194 (-137.675, 110.5) -> (-134.5, 113.675) centre (-137.675, 113.675) ccw
  line L195 (-137.675, 110.5) -> (-150.325, 110.5)
  arc A195 (-153.5, 113.675) -> (-150.325, 110.5) centre (-150.325, 113.675) ccw
  line L196 (-57.5, 113.675) -> (-57.5, 126.325)
  arc A196 (-54.325, 129.5) -> (-57.5, 126.325) centre (-54.325, 126.325) ccw
  line L197 (-54.325, 129.5) -> (-41.675, 129.5)
  arc A197 (-38.5, 126.325) -> (-41.675, 129.5) centre (-41.675, 126.325) ccw
  line L198 (-38.5, 126.325) -> (-38.5, 113.675)
  arc A198 (-41.675, 110.5) -> (-38.5, 113.675) centre (-41.675, 113.675) ccw
  line L199 (-41.675, 110.5) -> (-54.325, 110.5)
  arc A199 (-57.5, 113.675) -> (-54.325, 110.5) centre (-54.325, 113.675) ccw
  line L200 (-129.5, 137.675) -> (-129.5, 150.325)
  arc A200 (-126.325, 153.5) -> (-129.5, 150.325) centre (-126.325, 150.325) ccw
  line L201 (-126.325, 153.5) -> (-113.675, 153.5)
  arc A201 (-110.5, 150.325) -> (-113.675, 153.5) centre (-113.675, 150.325) ccw
  line L202 (-110.5, 150.325) -> (-110.5, 137.675)
  arc A202 (-113.675, 134.5) -> (-110.5, 137.675) centre (-113.675, 137.675) ccw
  line L203 (-113.675, 134.5) -> (-126.325, 134.5)
  arc A203 (-129.5, 137.675) -> (-126.325, 134.5) centre (-126.325, 137.675) ccw
  line L204 (-33.5, 137.675) -> (-33.5, 150.325)
  arc A204 (-30.325, 153.5) -> (-33.5, 150.325) centre (-30.325, 150.325) ccw
  line L205 (-30.325, 153.5) -> (-17.675, 153.5)
  arc A205 (-14.5, 150.325) -> (-17.675, 153.5) centre (-17.675, 150.325) ccw
  line L206 (-14.5, 150.325) -> (-14.5, 137.675)
  arc A206 (-17.675, 134.5) -> (-14.5, 137.675) centre (-17.675, 137.675) ccw
  line L207 (-17.675, 134.5) -> (-30.325, 134.5)
  arc A207 (-33.5, 137.675) -> (-30.325, 134.5) centre (-30.325, 137.675) ccw
  line L208 (-105.5, 161.675) -> (-105.5, 174.325)
  arc A208 (-102.325, 177.5) -> (-105.5, 174.325) centre (-102.325, 174.325) ccw
  line L209 (-102.325, 177.5) -> (-89.675, 177.5)
  arc A209 (-86.5, 174.325) -> (-89.675, 177.5) centre (-89.675, 174.325) ccw
  line L210 (-86.5, 174.325) -> (-86.5, 161.675)
  arc A210 (-89.675, 158.5) -> (-86.5, 161.675) centre (-89.675, 161.675) ccw
  line L211 (-89.675, 158.5) -> (-102.325, 158.5)
  arc A211 (-105.5, 161.675) -> (-102.325, 158.5) centre (-102.325, 161.675) ccw
  line L212 (86.5, -174.325) -> (86.5, -161.675)
  arc A212 (89.675, -158.5) -> (86.5, -161.675) centre (89.675, -161.675) ccw
  line L213 (89.675, -158.5) -> (102.325, -158.5)
  arc A213 (105.5, -161.675) -> (102.325, -158.5) centre (102.325, -161.675) ccw
  line L214 (105.5, -161.675) -> (105.5, -174.325)
  arc A214 (102.325, -177.5) -> (105.5, -174.325) centre (102.325, -174.325) ccw
  line L215 (102.325, -177.5) -> (89.675, -177.5)
  arc A215 (86.5, -174.325) -> (89.675, -177.5) centre (89.675, -174.325) ccw
  line L216 (134.5, -126.325) -> (134.5, -113.675)
  arc A216 (137.675, -110.5) -> (134.5, -113.675) centre (137.675, -113.675) ccw
  line L217 (137.675, -110.5) -> (150.325, -110.5)
  arc A217 (153.5, -113.675) -> (150.325, -110.5) centre (150.325, -113.675) ccw
  line L218 (153.5, -113.675) -> (153.5, -126.325)
  arc A218 (150.325, -129.5) -> (153.5, -126.325) centre (150.325, -126.325) ccw
  line L219 (150.325, -129.5) -> (137.675, -129.5)
  arc A219 (134.5, -126.325) -> (137.675, -129.5) centre (137.675, -126.325) ccw
  line L220 (86.5, -54.325) -> (86.5, -41.675)
  arc A220 (89.675, -38.5) -> (86.5, -41.675) centre (89.675, -41.675) ccw
  line L221 (89.675, -38.5) -> (102.325, -38.5)
  arc A221 (105.5, -41.675) -> (102.325, -38.5) centre (102.325, -41.675) ccw
  line L222 (105.5, -41.675) -> (105.5, -54.325)
  arc A222 (102.325, -57.5) -> (105.5, -54.325) centre (102.325, -54.325) ccw
  line L223 (102.325, -57.5) -> (89.675, -57.5)
  arc A223 (86.5, -54.325) -> (89.675, -57.5) centre (89.675, -54.325) ccw
  line L224 (-177.5, 41.675) -> (-177.5, 54.325)
  arc A224 (-174.325, 57.5) -> (-177.5, 54.325) centre (-174.325, 54.325) ccw
  line L225 (-174.325, 57.5) -> (-161.675, 57.5)
  arc A225 (-158.5, 54.325) -> (-161.675, 57.5) centre (-161.675, 54.325) ccw
  line L226 (-158.5, 54.325) -> (-158.5, 41.675)
  arc A226 (-161.675, 38.5) -> (-158.5, 41.675) centre (-161.675, 41.675) ccw
  line L227 (-161.675, 38.5) -> (-174.325, 38.5)
  arc A227 (-177.5, 41.675) -> (-174.325, 38.5) centre (-174.325, 41.675) ccw
  line L228 (110.5, -54.325) -> (110.5, -41.675)
  arc A228 (113.675, -38.5) -> (110.5, -41.675) centre (113.675, -41.675) ccw
  line L229 (113.675, -38.5) -> (126.325, -38.5)
  arc A229 (129.5, -41.675) -> (126.325, -38.5) centre (126.325, -41.675) ccw
  line L230 (129.5, -41.675) -> (129.5, -54.325)
  arc A230 (126.325, -57.5) -> (129.5, -54.325) centre (126.325, -54.325) ccw
  line L231 (126.325, -57.5) -> (113.675, -57.5)
  arc A231 (110.5, -54.325) -> (113.675, -57.5) centre (113.675, -54.325) ccw
  line L232 (158.5, -126.325) -> (158.5, -113.675)
  arc A232 (161.675, -110.5) -> (158.5, -113.675) centre (161.675, -113.675) ccw
  line L233 (161.675, -110.5) -> (174.325, -110.5)
  arc A233 (177.5, -113.675) -> (174.325, -110.5) centre (174.325, -113.675) ccw
  line L234 (177.5, -113.675) -> (177.5, -126.325)
  arc A234 (174.325, -129.5) -> (177.5, -126.325) centre (174.325, -126.325) ccw
  line L235 (174.325, -129.5) -> (161.675, -129.5)
  arc A235 (158.5, -126.325) -> (161.675, -129.5) centre (161.675, -126.325) ccw
  line L236 (110.5, -174.325) -> (110.5, -161.675)
  arc A236 (113.675, -158.5) -> (110.5, -161.675) centre (113.675, -161.675) ccw
  line L237 (113.675, -158.5) -> (126.325, -158.5)
  arc A237 (129.5, -161.675) -> (126.325, -158.5) centre (126.325, -161.675) ccw
  line L238 (129.5, -161.675) -> (129.5, -174.325)
  arc A238 (126.325, -177.5) -> (129.5, -174.325) centre (126.325, -174.325) ccw
  line L239 (126.325, -177.5) -> (113.675, -177.5)
  arc A239 (110.5, -174.325) -> (113.675, -177.5) centre (113.675, -174.325) ccw
  line L240 (-81.5, 161.675) -> (-81.5, 174.325)
  arc A240 (-78.325, 177.5) -> (-81.5, 174.325) centre (-78.325, 174.325) ccw
  line L241 (-78.325, 177.5) -> (-65.675, 177.5)
  arc A241 (-62.5, 174.325) -> (-65.675, 177.5) centre (-65.675, 174.325) ccw
  line L242 (-62.5, 174.325) -> (-62.5, 161.675)
  arc A242 (-65.675, 158.5) -> (-62.5, 161.675) centre (-65.675, 161.675) ccw
  line L243 (-65.675, 158.5) -> (-78.325, 158.5)
  arc A243 (-81.5, 161.675) -> (-78.325, 158.5) centre (-78.325, 161.675) ccw
  line L244 (-177.5, 161.675) -> (-177.5, 174.325)
  arc A244 (-174.325, 177.5) -> (-177.5, 174.325) centre (-174.325, 174.325) ccw
  line L245 (-174.325, 177.5) -> (-161.675, 177.5)
  arc A245 (-158.5, 174.325) -> (-161.675, 177.5) centre (-161.675, 174.325) ccw
  line L246 (-158.5, 174.325) -> (-158.5, 161.675)
  arc A246 (-161.675, 158.5) -> (-158.5, 161.675) centre (-161.675, 161.675) ccw
  line L247 (-161.675, 158.5) -> (-174.325, 158.5)
  arc A247 (-177.5, 161.675) -> (-174.325, 158.5) centre (-174.325, 161.675) ccw
  line L248 (-105.5, 137.675) -> (-105.5, 150.325)
  arc A248 (-102.325, 153.5) -> (-105.5, 150.325) centre (-102.325, 150.325) ccw
  line L249 (-102.325, 153.5) -> (-89.675, 153.5)
  arc A249 (-86.5, 150.325) -> (-89.675, 153.5) centre (-89.675, 150.325) ccw
  line L250 (-86.5, 150.325) -> (-86.5, 137.675)
  arc A250 (-89.675, 134.5) -> (-86.5, 137.675) centre (-89.675, 137.675) ccw
  line L251 (-89.675, 134.5) -> (-102.325, 134.5)
  arc A251 (-105.5, 137.675) -> (-102.325, 134.5) centre (-102.325, 137.675) ccw
  line L252 (-33.5, 113.675) -> (-33.5, 126.325)
  arc A252 (-30.325, 129.5) -> (-33.5, 126.325) centre (-30.325, 126.325) ccw
  line L253 (-30.325, 129.5) -> (-17.675, 129.5)
  arc A253 (-14.5, 126.325) -> (-17.675, 129.5) centre (-17.675, 126.325) ccw
  line L254 (-14.5, 126.325) -> (-14.5, 113.675)
  arc A254 (-17.675, 110.5) -> (-14.5, 113.675) centre (-17.675, 113.675) ccw
  line L255 (-17.675, 110.5) -> (-30.325, 110.5)
  arc A255 (-33.5, 113.675) -> (-30.325, 110.5) centre (-30.325, 113.675) ccw
  line L256 (-129.5, 113.675) -> (-129.5, 126.325)
  arc A256 (-126.325, 129.5) -> (-129.5, 126.325) centre (-126.325, 126.325) ccw
  line L257 (-126.325, 129.5) -> (-113.675, 129.5)
  arc A257 (-110.5, 126.325) -> (-113.675, 129.5) centre (-113.675, 126.325) ccw
  line L258 (-110.5, 126.325) -> (-110.5, 113.675)
  arc A258 (-113.675, 110.5) -> (-110.5, 113.675) centre (-113.675, 113.675) ccw
  line L259 (-113.675, 110.5) -> (-126.325, 110.5)
  arc A259 (-129.5, 113.675) -> (-126.325, 110.5) centre (-126.325, 113.675) ccw
  line L260 (-57.5, 89.675) -> (-57.5, 102.325)
  arc A260 (-54.325, 105.5) -> (-57.5, 102.325) centre (-54.325, 102.325) ccw
  line L261 (-54.325, 105.5) -> (-41.675, 105.5)
  arc A261 (-38.5, 102.325) -> (-41.675, 105.5) centre (-41.675, 102.325) ccw
  line L262 (-38.5, 102.325) -> (-38.5, 89.675)
  arc A262 (-41.675, 86.5) -> (-38.5, 89.675) centre (-41.675, 89.675) ccw
  line L263 (-41.675, 86.5) -> (-54.325, 86.5)
  arc A263 (-57.5, 89.675) -> (-54.325, 86.5) centre (-54.325, 89.675) ccw
  line L264 (-153.5, 89.675) -> (-153.5, 102.325)
  arc A264 (-150.325, 105.5) -> (-153.5, 102.325) centre (-150.325, 102.325) ccw
  line L265 (-150.325, 105.5) -> (-137.675, 105.5)
  arc A265 (-134.5, 102.325) -> (-137.675, 105.5) centre (-137.675, 102.325) ccw
  line L266 (-134.5, 102.325) -> (-134.5, 89.675)
  arc A266 (-137.675, 86.5) -> (-134.5, 89.675) centre (-137.675, 89.675) ccw
  line L267 (-137.675, 86.5) -> (-150.325, 86.5)
  arc A267 (-153.5, 89.675) -> (-150.325, 86.5) centre (-150.325, 89.675) ccw
  line L268 (-81.5, 65.675) -> (-81.5, 78.325)
  arc A268 (-78.325, 81.5) -> (-81.5, 78.325) centre (-78.325, 78.325) ccw
  line L269 (-78.325, 81.5) -> (-65.675, 81.5)
  arc A269 (-62.5, 78.325) -> (-65.675, 81.5) centre (-65.675, 78.325) ccw
  line L270 (-62.5, 78.325) -> (-62.5, 65.675)
  arc A270 (-65.675, 62.5) -> (-62.5, 65.675) centre (-65.675, 65.675) ccw
  line L271 (-65.675, 62.5) -> (-78.325, 62.5)
  arc A271 (-81.5, 65.675) -> (-78.325, 62.5) centre (-78.325, 65.675) ccw
  line L272 (-177.5, 65.675) -> (-177.5, 78.325)
  arc A272 (-174.325, 81.5) -> (-177.5, 78.325) centre (-174.325, 78.325) ccw
  line L273 (-174.325, 81.5) -> (-161.675, 81.5)
  arc A273 (-158.5, 78.325) -> (-161.675, 81.5) centre (-161.675, 78.325) ccw
  line L274 (-158.5, 78.325) -> (-158.5, 65.675)
  arc A274 (-161.675, 62.5) -> (-158.5, 65.675) centre (-161.675, 65.675) ccw
  line L275 (-161.675, 62.5) -> (-174.325, 62.5)
  arc A275 (-177.5, 65.675) -> (-174.325, 62.5) centre (-174.325, 65.675) ccw
  line L276 (-129.5, -78.325) -> (-129.5, -65.675)
  arc A276 (-126.325, -62.5) -> (-129.5, -65.675) centre (-126.325, -65.675) ccw
  line L277 (-126.325, -62.5) -> (-113.675, -62.5)
  arc A277 (-110.5, -65.675) -> (-113.675, -62.5) centre (-113.675, -65.675) ccw
  line L278 (-110.5, -65.675) -> (-110.5, -78.325)
  arc A278 (-113.675, -81.5) -> (-110.5, -78.325) centre (-113.675, -78.325) ccw
  line L279 (-113.675, -81.5) -> (-126.325, -81.5)
  arc A279 (-129.5, -78.325) -> (-126.325, -81.5) centre (-126.325, -78.325) ccw
  line L280 (-153.5, -102.325) -> (-153.5, -89.675)
  arc A280 (-150.325, -86.5) -> (-153.5, -89.675) centre (-150.325, -89.675) ccw
  line L281 (-150.325, -86.5) -> (-137.675, -86.5)
  arc A281 (-134.5, -89.675) -> (-137.675, -86.5) centre (-137.675, -89.675) ccw
  line L282 (-134.5, -89.675) -> (-134.5, -102.325)
  arc A282 (-137.675, -105.5) -> (-134.5, -102.325) centre (-137.675, -102.325) ccw
  line L283 (-137.675, -105.5) -> (-150.325, -105.5)
  arc A283 (-153.5, -102.325) -> (-150.325, -105.5) centre (-150.325, -102.325) ccw
  line L284 (-177.5, -126.325) -> (-177.5, -113.675)
  arc A284 (-174.325, -110.5) -> (-177.5, -113.675) centre (-174.325, -113.675) ccw
  line L285 (-174.325, -110.5) -> (-161.675, -110.5)
  arc A285 (-158.5, -113.675) -> (-161.675, -110.5) centre (-161.675, -113.675) ccw
  line L286 (-158.5, -113.675) -> (-158.5, -126.325)
  arc A286 (-161.675, -129.5) -> (-158.5, -126.325) centre (-161.675, -126.325) ccw
  line L287 (-161.675, -129.5) -> (-174.325, -129.5)
  arc A287 (-177.5, -126.325) -> (-174.325, -129.5) centre (-174.325, -126.325) ccw
  line L288 (-129.5, -174.325) -> (-129.5, -161.675)
  arc A288 (-126.325, -158.5) -> (-129.5, -161.675) centre (-126.325, -161.675) ccw
  line L289 (-126.325, -158.5) -> (-113.675, -158.5)
  arc A289 (-110.5, -161.675) -> (-113.675, -158.5) centre (-113.675, -161.675) ccw
  line L290 (-110.5, -161.675) -> (-110.5, -174.325)
  arc A290 (-113.675, -177.5) -> (-110.5, -174.325) centre (-113.675, -174.325) ccw
  line L291 (-113.675, -177.5) -> (-126.325, -177.5)
  arc A291 (-129.5, -174.325) -> (-126.325, -177.5) centre (-126.325, -174.325) ccw
  line L292 (14.5, -150.325) -> (14.5, -137.675)
  arc A292 (17.675, -134.5) -> (14.5, -137.675) centre (17.675, -137.675) ccw
  line L293 (17.675, -134.5) -> (30.325, -134.5)
  arc A293 (33.5, -137.675) -> (30.325, -134.5) centre (30.325, -137.675) ccw
  line L294 (33.5, -137.675) -> (33.5, -150.325)
  arc A294 (30.325, -153.5) -> (33.5, -150.325) centre (30.325, -150.325) ccw
  line L295 (30.325, -153.5) -> (17.675, -153.5)
  arc A295 (14.5, -150.325) -> (17.675, -153.5) centre (17.675, -150.325) ccw
  line L296 (-33.5, -54.325) -> (-33.5, -41.675)
  arc A296 (-30.325, -38.5) -> (-33.5, -41.675) centre (-30.325, -41.675) ccw
  line L297 (-30.325, -38.5) -> (-17.675, -38.5)
  arc A297 (-14.5, -41.675) -> (-17.675, -38.5) centre (-17.675, -41.675) ccw
  line L298 (-14.5, -41.675) -> (-14.5, -54.325)
  arc A298 (-17.675, -57.5) -> (-14.5, -54.325) centre (-17.675, -54.325) ccw
  line L299 (-17.675, -57.5) -> (-30.325, -57.5)
  arc A299 (-33.5, -54.325) -> (-30.325, -57.5) centre (-30.325, -54.325) ccw
  line L300 (14.5, -174.325) -> (14.5, -161.675)